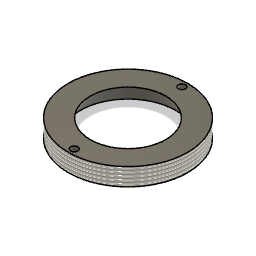
Collet Top Taper v1 (Autodesk Fusion 360 design; units mm, degrees)
Autodesk Fusion 360 part; units mm, degrees
sketch "Sketch1" plane through (0, 0, 0) normal (0, 0, 1) x (1, 0, 0)
  line L0 (-20.7744, 0) -> (-26.35, 0)
  line L1 (-26.35, 0) -> (-26.35, 7.62)
  line L2 (-26.35, 7.62) -> (-16.375, 7.62)
  line L3 (-16.375, 7.62) -> (-20.7744, 0)
  dimension "d1" = 26.35
  dimension "d2" = 16.375
  dimension "d3" = 60
  dimension "d4" = 7.62
  dimension "d5" = 7.62
  constraint horizontal L0
  constraint perpendicular L0 L1
  constraint perpendicular L1 L2
  measures "d1" horizontal distance of origin L0.end
  measures "d2" horizontal distance of origin L2.end
  measures "d3" angle of L0 L3
  measures "d4" vertical distance of L0.end L1.end
  measures "d5" vertical distance of origin L2.end
sketch "Sketch2" plane through (0, 0, 0) normal (0, 0, 1) x (1, 0, 0)
  line L0 (0, 0) -> (0, 1)
  line L1 (0, 1) -> (0, 14) construction
  constraint coincident L0.start origin
  constraint vertical L0
  constraint parallel L0 L1
revolve "Revolve1" add sketch "Sketch1" angle 360 about axis through (0, 1, 0) along (0, 1, 0)
thread "Thread1" "ISO Metric profile 52.0 M52x1.5 6g" major diameter 51.85 minor diameter 50.1269 pitch 1.5 angle 60 resizes the face on face at (-26.2191, 2.54, -2.6236)
sketch "Sketch3" plane through (0, 7.62, 0) normal (0, 1, 0) x (-1, 0, 0)
  circle A0 centre (0, 0) radius 25.925
  circle A1 centre (0, 0) radius 16.375
  point P0 (-0.0141, -23.35)
  point P1 (-0.0141, 23.35)
  dimension "d7" = 46.7
  dimension "d8" = 23.35
  measures "d7" vertical distance of P0 P1
  measures "d8" vertical distance of A0.centre P0
hole "Hole1" at (0.0141, 7.62, -23.35) at (0.0141, 7.62, 23.35) direction (0, -1, 0) diameter 3.1 depth 13.5 tip angle 118
equation "d1 = ( 52.7 / 2 ) * 1 mm"
equation "d2 = ( 32.75 / 2 ) * 1 mm"
